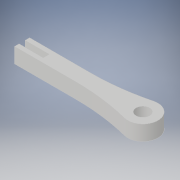
# Autodesk Inventor part: ChipPusher
Saved by Autodesk Inventor 2019 (Build 230136000, 136)
## iProperties
Created: 2019-06-14
Part Number: ChipPusher
Material: Generic
Document SubType Name: Modeling
Designer: aorfi
Density: 1 g/cm^3
Appearance: Default
Author: aorfi
Autodesk Inventor part; units mm, degrees
ref_plane "YZ Plane" through (0, 0, 0) normal (1, 0, 0) x (0, 1, 0)
ref_plane "XZ Plane" through (0, 0, 0) normal (0, 1, 0) x (-1, 0, 0)
ref_plane "XY Plane" through (0, 0, 0) normal (0, 0, 1) x (1, 0, 0)
sketch "Sketch1" plane through (0, 0, 0) normal (0, 1, 0) x (-1, 0, 0)
  line L0 (-10, 2.5) -> (10, 2.5)
  line L1 (10, 2.5) -> (10, -2.5)
  line L2 (10, -2.5) -> (-10, -2.5)
  line L3 (-10, -2.5) -> (-10, 2.5)
  line L4 (-10, 2.5) -> (10, -2.5) construction
  line L5 (10, 2.5) -> (-10, -2.5) construction
  line L6 (10, 1) -> (2, 1)
  line L7 (2, 1) -> (2, -1)
  line L8 (2, -1) -> (10, -1)
  line L9 (10, -1) -> (10, 1)
  circle A0 centre (-30, 0) radius 5
  arc A1 (-10, -2.5) -> (-28.7692, -4.8462) centre (-10, -78.75) ccw
  arc A2 (-28.7692, 4.8462) -> (-10, 2.5) centre (-10, 78.75) ccw
  point P0 (0, 0)
  point P1 (0, 0)
  point P2 (2, 0)
  point P3 (0, 0)
  dimension "d0" = 5
  dimension "d1" = 20
  dimension "d2" = 8
  dimension "d3" = 2
  dimension "d6" = 10
  dimension "d7" = 30
  constraints: 21 end point, 6 point on circle, 5 midpoint, 4 parallel, 4 tangent, 3 centre point, 2 horizontal, 2 horizontal alignment, 2 perpendicular, 1 point on line
  measures "d0" distance of L0.end L1.end
  measures "d1" distance of L1.end L2.end
  measures "d2" distance of L6.start L6.end
  measures "d3" distance of L6.end L7.end
  measures "d6" diameter of A0
  measures "d7" distance of A0.centre point (0, 0)
extrude "Extrusion1" add sketch "Sketch1" along normal mid plane 5 contours L0 L1 L6 L7 L8 L2 L3 | L3 A1 A0 A2 | A0
sketch "Sketch3" plane through (0, 2.5, 0) normal (0, 1, 0) x (1, 0, 0)
  arc A0 (28.7692, -4.8462) -> (28.7692, -4.8462) centre (30, 0) ccw projected
  point P0 (0, 0)
  point P1 (37.473, -9.6754)
  point P2 (37.473, 9.6754)
  point P3 (23.4247, 7.5342)
  constraints: 1 other
hole "Hole1" at (30, 2.5, 0) direction (0, -1, 0) diameter 4.496 end through all
body "Solid1"
